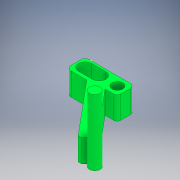
# Autodesk Inventor part: finger_4_slim
Saved by Autodesk Inventor 2018 (Build 220112000, 112)
## iProperties
Created: 2019-01-07
Part Number: finger_4_slim
Material: 一般
Document SubType Name: Modeling
Designer: lowyu
Density: 1 g/cm^3
Appearance: 既定
Author: lowyu
Autodesk Inventor part; units mm, degrees
ref_plane "YZ Plane" through (0, 0, 0) normal (1, 0, 0) x (0, 1, 0)
ref_plane "XZ Plane" through (0, 0, 0) normal (0, 1, 0) x (-1, 0, 0)
ref_plane "XY Plane" through (0, 0, 0) normal (0, 0, 1) x (1, 0, 0)
sketch "スケッチ1" plane through (0, 0, 0) normal (0, 0, 1) x (1, 0, 0)
  line L0 (18.4549, -8.1589) -> (14.4552, -8.1589)
  arc A0 (18.4549, -8.1589) -> (20.0703, -6.5435) centre (18.4549, -6.5435) ccw
  line L1 (20.0703, -2.0624) -> (20.0703, -6.5435)
  line L2 (18.0495, -0.0417) -> (-1.0589, -0.0417)
  arc A1 (-1.0589, -0.0417) -> (-2.9016, -1.8843) centre (-1.0589, -1.8843) ccw
  line L3 (-2.9016, -1.8843) -> (-2.9016, -6.5559)
  arc A2 (-2.9016, -6.5559) -> (-0.7003, -8.7571) centre (-0.7003, -6.5559) ccw
  arc A3 (26.8987, -33.0319) -> (28.4367, -33.0608) centre (27.7277, -29.8571) ccw
  line L4 (30.1493, -31.6136) -> (28.4367, -33.0608)
  arc A4 (30.1493, -31.6136) -> (31.6494, -28.7162) centre (32.5816, -31.0359) ccw
  line L5 (31.6494, -28.7162) -> (14.4552, -8.1589)
  circle A5 centre (16.1123, -4.0657) radius 2.5
  line L6 (7.6373, -0.9827) -> (1.1644, -0.9827)
  arc A6 (7.6373, -7.2327) -> (7.6373, -0.9827) centre (7.6373, -4.1077) ccw
  arc A7 (1.1644, -0.9827) -> (1.1644, -7.2327) centre (1.1644, -4.1077) ccw
  line L7 (26.8987, -33.0319) -> (6.5951, -8.7571)
  line L8 (-0.7003, -8.7571) -> (6.5951, -8.7571)
  arc A8 (20.0703, -2.0624) -> (18.0495, -0.0417) centre (18.0495, -2.0624) ccw
  line L9 (1.1644, -7.2327) -> (7.6373, -7.2327)
  line L10 (13.6123, -4.0657) -> (13.6123, 1.3375)
  line L11 (10.7623, -4.0657) -> (10.7623, 0.9924)
  point P0 (0, 0)
  dimension "d0" = 5
  dimension "d1" = 3.125
  dimension "d17" = 4.8539
  dimension "d44" = 4.066
  dimension "d45" = 4.066
  dimension "d46" = 90
  dimension "d47" = 90
  dimension "d48" = 3.125
  dimension "d53" = 3.9579
  dimension "d54" = 22.9718
  dimension "d62" = 2.5
  dimension "d63" = 2.85
  constraints: 24 end point, 16 point on circle, 11 tangent, 8 centre point, 4 parallel, 2 horizontal, 2 perpendicular, 1 coincident, 1 horizontal alignment, 1 vertical, 2 other
  measures "d1" radius of A6
  measures "d17" horizontal distance of A4.centre A3.centre
  measures "d44" distance from line of L2 A7.centre
  measures "d45" distance from line of L3 A7.centre
  measures "d48" radius of A7
  measures "d53" distance from line of L1 point (16.112, -4.066)
  measures "d54" distance between parallel lines of L1 L3
  measures "d62" radius of A4
  measures "d63" distance between parallel lines of L10 L11
extrude "押し出し1" add sketch "スケッチ1" along normal blind 10.6
sketch "スケッチ2" plane through (0, 0, 10.6) normal (0, 0, 1) x (1, 0, 0)
  point P0 (0, 0)
sketch "スケッチ3" plane through (0, 0, 10.6) normal (0, 0, 1) x (1, 0, 0)
  arc A0 (30.1493, -31.6136) -> (31.6494, -28.7162) centre (32.5816, -31.0359) ccw projected
  arc A1 (31.6494, -28.7162) -> (30.1493, -31.6136) centre (32.5816, -31.0359) ccw
  point P0 (0, 0)
  constraints: 2 point on circle, 1 centre point, 1 coincident
extrude "押し出し2" add sketch "スケッチ3" along normal blind 20
equation "\"d45\" = d44"
equation "\"d48\" = d1"
